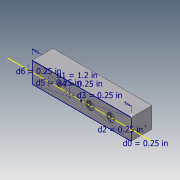
# Autodesk Inventor part: J010309
Saved by Autodesk Inventor 2020.4 (Build 244396000, 396)
## iProperties
RuleStatus: InUse
AfterDocSave0: file://Part Number Cleaner
Created: 2022-04-27
Material: ALUMINUM, 6061-T651
Catalog Web Link: https://www.janelia.org/
Vendor: HHMI: JRC - JET
Document SubType Name: Modeling
Designer: arnoldj
Density: 2.7 g/cm^3
Appearance: Metal-AL-6061 (Machined)
Part Number: J010309
Project: COMMON
Description: VP SPRING HOLDER
LAB/DEPT: COMMON
REQUESTING SCIENTIST: COMMON
SURFACE ROUGHNESS: N/A
DESIGN DEPARTMENT: HHMI: JRC - ID&F
SPECIAL FINISH: NONE
ALTERED ITEM PART NUMBER: N/A
ALTERED ITEM VENDOR: N/A
ALTERED ITEM DESCRIPTION: N/A
Title: Standard
Author: arnoldj
Revision Number: -
Autodesk Inventor part; units mm, degrees
ref_plane "YZ Plane" through (0, 0, 0) normal (1, 0, 0) x (0, 1, 0)
ref_plane "XZ Plane" through (0, 0, 0) normal (0, 1, 0) x (-1, 0, 0)
ref_plane "XY Plane" through (0, 0, 0) normal (0, 0, 1) x (1, 0, 0)
sketch "Sketch1" plane through (0, 0, 0) normal (0, 0, 1) x (1, 0, 0)
  line L0 (0, 4.445) -> (0, -4.445) projected
  line L1 (-38.1, 0) -> (6.35, 0) projected
  line L2 (-30.48, -3.175) -> (0, -3.175)
  line L3 (0, -3.175) -> (0, 3.175)
  line L4 (0, 3.175) -> (-30.48, 3.175)
  line L5 (-30.48, 3.175) -> (-30.48, -3.175)
  line L6 (-30.48, -3.175) -> (0, 3.175) construction
  line L7 (0, -3.175) -> (-30.48, 3.175) construction
  point P0 (0, 0)
  point P1 (-15.24, 0)
  point P2 (-6.35, 0)
  point P3 (-12.7, 0)
  point P4 (-19.05, 0)
  point P5 (-25.4, 0)
  point P6 (-31.75, 0)
  dimension "d0" = 6.35
  dimension "d1" = 30.48
  dimension "d2" = 6.35
  dimension "d3" = 6.35
  dimension "d4" = 6.35
  dimension "d5" = 6.35
  dimension "d6" = 6.35
  constraints: 12 end point, 2 midpoint, 2 parallel, 1 horizontal, 1 perpendicular, 1 point on line, 7 other
  measures "d0" distance between parallel lines of L2 L4
  measures "d1" distance of L3.end L4.end
  measures "d2" distance from line of point (-6.35, 0) L0
  measures "d3" distance of point (-6.35, 0) point (-12.7, 0)
  measures "d4" distance of point (-12.7, 0) point (-19.05, 0)
  measures "d5" distance of point (-19.05, 0) point (-25.4, 0)
  measures "d6" distance of point (-25.4, 0) point (-31.75, 0)
extrude "Extrusion1" add sketch "Sketch1" against normal blind 6.35
hole "Hole1" at (-6.35, 0, 0) at (-12.7, 0, 0) direction (0, 0, -1) diameter 2.6416 end through all thread size "6-32 UNC" class "2B" standard "ANSI Unified Screw Threads"
hole "Hole2" [suppressed]
fillet "Fillet1" [suppressed]
sketch "Sketch2" plane through (-30.48, -3.175, 0) normal (-1, 0, 0) x (0, 0, 1)
  line L0 (0, 6.35) -> (0, 0) projected
  line L1 (0, 6.35) -> (-6.35, 6.35) projected
  line L2 (-6.35, 0) -> (-6.35, 6.35) projected
  line L3 (0, 0) -> (-6.35, 0) projected
  line L4 (-6.35, 0) -> (-6.35, 6.35) construction
  line L5 (-6.35, 6.35) -> (0, 0) construction
  point P0 (0, 3.175)
  point P1 (-3.175, 3.175)
  constraints: 2 end point, 1 midpoint
hole "Hole3" at (-30.48, 0, -3.175) direction (1, 0, 0) diameter 3.302 depth 12.7 tip angle 118 thread size "8-32 UNC" class "2B" standard "ANSI Unified Screw Threads"
body "Solid1"
